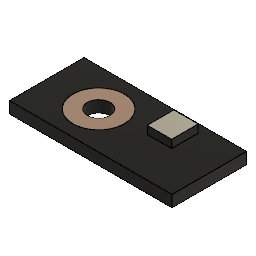
extruder_body_bltouch_190604 (Autodesk Fusion 360 archive; units mm, degrees)
design "filament_sensor"
Autodesk Fusion 360 part; units mm, degrees
sketch "Sketch1" plane through (0, 0, 0) normal (0, 0, 1) x (1, 0, 0)
  line L0 (0, 0) -> (22.2, 0)
  line L1 (22.2, 0) -> (22.2, 10.2)
  line L2 (22.2, 10.2) -> (0, 10.2)
  line L3 (0, 10.2) -> (0, 0)
  circle A0 centre (7.1, 5.1) radius 1.55
  line L4 (13.45, 9) -> (16.75, 9)
  line L5 (16.75, 9) -> (16.75, 5.4)
  line L6 (16.75, 5.4) -> (13.45, 5.4)
  line L7 (13.45, 5.4) -> (13.45, 9)
  circle A1 centre (7.1, 5.1) radius 3.5
  line L8 (15.1, 9) -> (15.1, 5.4) construction
  line L9 (11.15, 9.8) -> (13.25, 9.8)
  line L10 (13.25, 9.8) -> (13.25, 5.6)
  line L11 (13.25, 5.6) -> (11.15, 5.6)
  line L12 (11.15, 5.6) -> (11.15, 9.8)
  line L13 (12.2, 9.8) -> (12.2, 5.6) construction
  dimension "d1" = 22.2
  dimension "d2" = 10.2
  dimension "d3" = 3.1
  dimension "d4" = 7
  dimension "d5" = 8
  dimension "d6" = 3.3
  dimension "d7" = 3.6
  dimension "d8" = 5.1
  dimension "d9" = 7.1
  dimension "d10" = 1.2
  dimension "d11" = 0.4
  dimension "d12" = 2.1
  dimension "d13" = 4.2
  dimension "d14" = 5.1
  measures "d2" distance of L0.start
  measures "d3" diameter of A0
  measures "d4" diameter of A1
  measures "d6" distance of L5 L7
  measures "d8" distance of L2
  measures "d9" distance of L3
  measures "d10" distance of L2 L4
  measures "d11" distance of L2 L9
  measures "d12" distance of L10 L12
  measures "d14" distance of L13
extrude "Extrude1" add sketch "Sketch1" against normal blind 1.6 contours L0 L1 L2 L3 | L4 L5 L6 L7 | A1 | L9 L10 L11 L12
extrude "Extrude2" add sketch "Sketch1" along normal blind 0.01 contours A1
extrude "Extrude3" add sketch "Sketch1" along normal blind 1.1 contours L4 L5 L6 L7

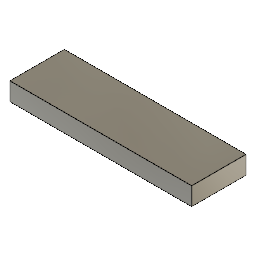
design "magnet_20x6x2"
Autodesk Fusion 360 part; units mm, degrees
sketch "Sketch1" plane through (0, 0, 0) normal (0, 0, 1) x (1, 0, 0)
  line L0 (0, 0) -> (20, 0)
  line L1 (20, 0) -> (20, 6)
  line L2 (20, 6) -> (0, 6)
  line L3 (0, 6) -> (0, 0)
  dimension "d1" = 6
  dimension "d2" = 20
  measures "d1" distance of L0.start
  measures "d2" distance of L0.start
extrude "Extrude1" add sketch "Sketch1" along normal blind 2

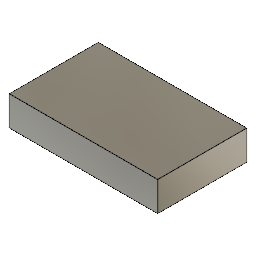
design "magnet_10x6x2"
Autodesk Fusion 360 part; units mm, degrees
sketch "Sketch1" plane through (0, 0, 0) normal (0, 0, 1) x (1, 0, 0)
  line L0 (0, 0) -> (10, 0)
  line L1 (10, 0) -> (10, 6)
  line L2 (10, 6) -> (0, 6)
  line L3 (0, 6) -> (0, 0)
  dimension "d1" = 10
  dimension "d2" = 6
  measures "d1" distance of L0.start
  measures "d2" distance of L0.start
extrude "Extrude1" add sketch "Sketch1" along normal blind 2

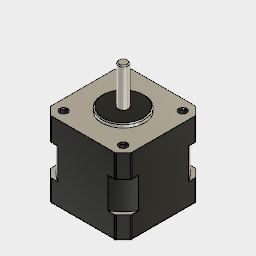
design "nema17_xye_ldo"
Autodesk Fusion 360 part; units mm, degrees
sketch "base" plane through (0, 0, 0) normal (0, 0, 1) x (1, 0, 0)
  line L0 (-21, -21) -> (21, -21)
  line L1 (21, -21) -> (21, 21)
  line L2 (21, 21) -> (-21, 21)
  line L3 (-21, 21) -> (-21, -21)
  line L4 (-21, -21) -> (21, 21) construction
  line L5 (21, -21) -> (-21, 21) construction
  circle A0 centre (0, 0) radius 11
  circle A1 centre (0, 0) radius 2.5
  circle A2 centre (-15.5, 15.5) radius 1.5
  circle A3 centre (15.5, 15.5) radius 1.5
  line L6 (-15.5, 15.5) -> (15.5, 15.5) construction
  circle A4 centre (15.5, -15.5) radius 1.5
  circle A5 centre (-15.5, -15.5) radius 1.5
  line L7 (-1.5, 2) -> (1.5, 2)
  dimension "d1" = 42
  dimension "d2" = 42
  dimension "d5" = 22
  dimension "d9" = 5
  dimension "d14" = 31
  dimension "d15" = 3
  dimension "d16" = 3
  dimension "d46" = 4.5
  measures "d1" distance of L0.end L1.end
  measures "d2" distance of L1.end L2.end
  measures "d5" diameter of A0
  measures "d9" diameter of A1
  measures "d14" distance of A2.centre A3.centre
  measures "d15" diameter of A2
  measures "d16" diameter of A3
extrude "Extrude1" add sketch "base" along normal blind 40 contours L0 L1 L2 L3 | A0 | A1 L7 | A1 L7 | A2 | A3 | A4 | A5 makes body 1
extrude "Extrude2" add sketch "base" along normal blind 2 from surface at 40 contours A0 | A1 L7 | A1 L7 bodies 1
extrude "Extrude3" add sketch "base" along normal blind 20 from surface at 42 contours A1 L7 picked at (0.6865, -0.2754) bodies 1
extrude "Extrude11" add sketch "base" along normal blind 1 from surface at 42 contours A1 L7 picked at (-0.3999, 2.0645) bodies 1
chamfer "Chamfer1" distance 4.2 angle 45 4 edges at (21, -21, 20) (21, 21, 20) (-21, 21, 20) (-21, -21, 20) on bodies 1
extrude "Extrude4" cut sketch "base" against normal blind 4.5 from surface at 40 contours A2 | A3 | A4 | A5 bodies 1
chamfer "Chamfer3" distance 0.5 angle 45 1 edges at (0, -2.5, 62) on bodies 1
chamfer "Chamfer4" distance 0.5 angle 45 1 edges at (-10.2556, -3.9778, 42) on bodies 1
sketch "core_shape" plane through (0, 0, 0) normal (0, 0, -1) x (1, 0, 0)
  line L0 (-16.8, 21) -> (-21, 16.8)
  line L1 (-21, 16.8) -> (-21, -16.8)
  line L2 (-21, -16.8) -> (-16.8, -21)
  line L3 (-16.8, -21) -> (16.8, -21)
  line L4 (16.8, -21) -> (21, -16.8)
  line L5 (21, -16.8) -> (21, 16.8)
  line L6 (21, 16.8) -> (16.8, 21)
  line L7 (16.8, 21) -> (-16.8, 21)
  circle A0 centre (0, 0) radius 24.7286
  line L8 (16.8, 21) -> (21, 16.8)
  arc A1 (1.5, -2) -> (-1.5, -2) centre (0, 0) ccw
  dimension "d31" = 2
  measures "d31" distance of A0 L8
extrude "Extrude6" cut sketch "core_shape" against normal up to surface (16 mm away) from surface at -12 contours L0 L1 L7 A0 | L5 L6 L7 A0 L8 | L1 L2 L3 A0 | L3 L4 L5 A0 bodies 1
sketch "back" plane through (0, 0, 0) normal (0, 0, -1) x (1, 0, 0)
  line L0 (-16.8, 21) -> (-21, 16.8)
  line L1 (-21, 16.8) -> (-21, -16.8)
  line L2 (-21, -16.8) -> (-16.8, -21)
  line L3 (-16.8, -21) -> (16.8, -21)
  line L4 (16.8, -21) -> (21, -16.8)
  line L5 (21, -16.8) -> (21, 16.8)
  line L6 (21, 16.8) -> (16.8, 21)
  line L7 (16.8, 21) -> (-16.8, 21)
  circle A0 centre (0, 0) radius 10.5
  circle A1 centre (0, 0) radius 3.479
  circle A2 centre (-15.5, 15.5) radius 1.5
  circle A3 centre (15.5, 15.5) radius 1.5
  circle A4 centre (-15.5, -15.5) radius 1.5
  circle A5 centre (15.5, -15.5) radius 1.5
  circle A6 centre (-15.5, 15.5) radius 3
  circle A7 centre (-15.5, -15.5) radius 3
  circle A8 centre (15.5, -15.5) radius 3
  circle A9 centre (15.5, 15.5) radius 3
  circle A10 centre (-15.5, 15.5) radius 2.6
  circle A11 centre (15.5, 15.5) radius 2.6
  circle A12 centre (-15.5, -15.5) radius 2.6
  circle A13 centre (15.5, -15.5) radius 2.6
  dimension "d50" = 6.958
  dimension "d58" = 6
  dimension "d59" = 6
  dimension "d60" = 6
  dimension "d61" = 6
  dimension "d62" = 5.2
  dimension "d63" = 5.2
  dimension "d64" = 5.2
  dimension "d65" = 5.2
  measures "d50" diameter of A1
  measures "d58" diameter of A6
  measures "d59" diameter of A7
  measures "d60" diameter of A8
  measures "d61" diameter of A9
  measures "d62" diameter of A10
  measures "d63" diameter of A11
  measures "d64" diameter of A12
  measures "d65" diameter of A13
extrude "Extrude8" cut sketch "back" against normal blind 2 contours A1 bodies 1
fillet "Fillet3" radius 0.2 1 edges at (-3.2436, -1.2581, 0) on bodies 1
extrude "Extrude10" cut sketch "back" against normal blind 4 contours A6 bodies 1
fillet "Fillet4" radius 1 1 edges at (-17.9241, -14.5598, 0) on bodies 1
pattern_circular "C-Pattern1" count 4 over 360 about axis through (0, 0, 1.75) along (0, 0, 1) of "Extrude10", "Fillet4"
sketch "cables" plane through (0, 21, 0) normal (0, 1, 0) x (-1, 0, 0)
  line L0 (-16.8, 0) -> (16.8, 0)
  circle A0 centre (0.75, 1.35) radius 0.75
  circle A1 centre (-0.75, 1.35) radius 0.75
  line L1 (-0.75, 1.35) -> (0.75, 1.35) construction
  line L2 (0.75, 1.35) -> (0.75, 0) construction
  line L3 (-0.75, 1.35) -> (-0.75, 2.85) construction
  line L4 (-0.75, 2.85) -> (0.75, 2.85) construction
  line L5 (0.75, 2.85) -> (0.75, 1.35) construction
  circle A2 centre (-0.75, 2.85) radius 0.75
  circle A3 centre (0.75, 2.85) radius 0.75
  line L6 (-3.5, 0) -> (3.5, 0)
  line L7 (3.5, 0) -> (3.5, 4)
  line L8 (3.5, 4) -> (-3.5, 4)
  line L9 (-3.5, 4) -> (-3.5, 0)
  line L10 (16.8, 0) -> (-16.8, 0)
  line L11 (-3.5, 0.3) -> (3.5, 0.3)
  dimension "d23" = 1.5
  dimension "d25" = 1.35
  dimension "d27" = 0.75
  dimension "d30" = 1.5
  dimension "d38" = 7
  dimension "d39" = 3.5
  dimension "d40" = 4
  dimension "d45" = 0.3
  measures "d23" diameter of A1
  measures "d25" distance of A0.centre L2.end
  measures "d27" distance of origin L2.end
  measures "d30" distance of A1.centre L2.end
  measures "d38" distance of L6.start L6.end
  measures "d39" distance of origin L6.end
  measures "d40" distance of L6.start L8.end
  measures "d45" distance of L6.end L11.end
extrude "Extrude5" add sketch "cables" along normal blind 5 separate body contours A0 | A1 | A3 | A2 makes body 2
extrude "Extrude7" add sketch "cables" along normal blind 0.3 and the other way blind 1.3 contours L7 L8 L9 L11 | A0 A1 A2 A3 | A3 | A2 bodies 1 2
fillet "Fillet1" radius 1 24 edges at (-21, 0, 0) (-18.9, -18.9, 0) (0, -21, 0) (-18.9, 18.9, 0) (0, 21, 0) (18.9, 18.9, 0) (21, 0, 0) (18.9, -18.9, 0) (-21, -16.8, 34) (-16.8, -21, 34) (-16.8, -21, 6) (-21, -16.8, 6) (-21, 16.8, 6) (-16.8, 21, 6) (-21, 16.8, 34) (-16.8, 21, 34) (16.8, 21, 34) (16.8, 21, 6) (21, 16.8, 34) (21, 16.8, 6) (21, -16.8, 6) (16.8, -21, 6) (16.8, -21, 34) (21, -16.8, 34) on bodies 1
chamfer "Chamfer2" distance 0.6 angle 45 4 edges at (14.1015, 16.0424, 40) (14.1015, -14.9576, 40) (-16.8985, -14.9576, 40) (-16.8985, 16.0424, 40) on bodies 1
equation "d26 = d23"
equation "d27 = d30 / 2"
equation "d30 = d23"
equation "d39 = d38 / 2"
equation "d59 = d58"
equation "d60 = d58"
equation "d61 = d58"
equation "d63 = d62"
equation "d64 = d62"
equation "d65 = d62"

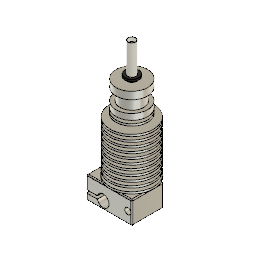
design "e3d_v6"
Autodesk Fusion 360 part; units mm, degrees
sketch "sink" plane through (0, 0, 0) normal (0, 0, 1) x (1, 0, 0) in component "sink"
  circle A0 centre (0, 0) radius 11.15
  circle A1 centre (0, 0) radius 6.4
  circle A2 centre (0, 0) radius 11
  dimension "d1" = 22.3
  dimension "d4" = 12.8
  dimension "d7" = 22
  dimension "d131" = 0
  dimension "d132" = 0
  dimension "d133" = 0
  dimension "d134" = 0
  dimension "d180" = 0
  dimension "d181" = 0
  dimension "d182" = 0
  dimension "d183" = 0
  dimension "d192" = 0
  dimension "d193" = 0
  dimension "d194" = 0
  dimension "d195" = 0
  constraint coincident A0.centre A1.centre
  constraint concentric A0 A1
  constraint concentric A1 A2
  measures "d1" diameter of A0
  measures "d4" diameter of A1
  measures "d7" diameter of A2
extrude "Extrude1" add sketch "sink" along normal blind 1 contours A0 | A1 | A2 makes body 1 in component "sink"
extrude "Extrude2" add sketch "sink" along normal blind 30 draft -3.6 contours A1 bodies 1 in component "sink"
extrude "Extrude3" add sketch "sink" along normal blind 1 from surface at 2.5 contours A1 | A2 bodies 1 in component "sink"
pattern_linear "R-Pattern1" count 10 spacing 2.5 along (0, 0, 1) of "Extrude3" in component "sink"
sketch "groove" plane through (0, 0, 30) normal (0, 0, 1) x (-1, 0, 0) in component "sink"
  circle A0 centre (0, 0) radius 4.5126
  circle A1 centre (0, 0) radius 4.5126
  circle A2 centre (0, 0) radius 8
  circle A3 centre (0, 0) radius 6
  dimension "d15" = 16
  dimension "d16" = 12
  constraint concentric A1 A2
  constraint concentric A2 A3
  measures "d15" diameter of A2
  measures "d16" diameter of A3
extrude "Extrude4" add sketch "groove" along normal blind 1 from surface at -2.5 contours A0 A1 | A2 | A3 bodies 1 in component "sink"
extrude "Extrude5" add sketch "groove" along normal blind 3 contours A0 A1 | A2 | A3 bodies 1 in component "sink"
extrude "Extrude6" add sketch "groove" along normal blind 6 from surface at 3 contours A0 A1 | A3 bodies 1 in component "sink"
extrude "Extrude7" add sketch "groove" along normal blind 3.7 from surface at 9 contours A0 A1 | A2 | A3 bodies 1 in component "sink"
sketch "top" plane through (0, 0, 42.7) normal (0, 0, 1) x (-1, 0, 0) in component "sink"
  circle A0 centre (0, 0) radius 8
  circle A1 centre (0, 0) radius 8
  circle A2 centre (0, 0) radius 3.5
  circle A3 centre (0, 0) radius 2.1
  circle A4 centre (0, 0) radius 2.5
  circle A5 centre (0, 0) radius 4
  dimension "d28" = 7
  dimension "d29" = 4.2
  dimension "d124" = 5
  dimension "d147" = 8
  constraint concentric A1 A2
  constraint concentric A2 A3
  constraint concentric A3 A4
  constraint concentric A4 A5
  measures "d28" diameter of A2
  measures "d29" diameter of A3
  measures "d124" diameter of A4
  measures "d147" diameter of A5
extrude "Extrude2'" cut sketch "top" against normal up to surface (42.7 mm away) contours A3 bodies 1 in component "sink"
extrude "Extrude3'" cut sketch "top" against normal blind 6.5 contours A2 | A4 | A5 bodies 1 in component "sink"
extrude "Extrude4'" cut sketch "top" against normal blind 2 draft -55 from surface at -6.5 contours A2 | A3 | A4 | A5 bodies 1 in component "sink"
extrude "Extrude5'" add sketch "top" against normal blind 6 contours A2 | A5 bodies 1 in component "sink"
extrude "Extrude8" add sketch "top" along normal blind 2 and the other way blind 5.5 contours A2 | A4 bodies 1 in component "sink"
extrude "Extrude1'" cut sketch "top" along normal blind 1 contours A2 bodies 1 in component "sink"
sketch "bottom" plane through (0, 0, 0) normal (0, 0, -1) x (1, 0, 0) in component "sink"
  circle A0 centre (0, 0) radius 2.1
  circle A1 centre (0, 0) radius 11.15
  circle A2 centre (0, 0) radius 3
  circle A3 centre (0, 0) radius 3.5
  dimension "d158" = 6
  dimension "d228" = 7
  constraint coincident A0.centre A1.centre
  constraint concentric A2 A3
  measures "d158" diameter of A2
  measures "d228" diameter of A3
extrude "Extrude6'" cut sketch "bottom" against normal blind 15.1 contours A0 | A2 bodies 1 in component "sink"
extrude "Extrude7'" cut sketch "bottom" against normal blind 2 draft -55 from surface at -15.1 contours A0 | A2 bodies 1 in component "sink"
extrude "Extrude8'" cut sketch "bottom" against normal blind 10.5 contours A3 bodies 1 in component "sink"
thread "Thread1" "ISO Metric profile 7.0 M7x1 6H" major diameter 7.1472 minor diameter 6.0355 pitch 1 angle 60 resizes the face on face at (3.4956, 0.1745, 7) on bodies 1 in component "sink"
sketch "Sketch4" plane through (0, 0, 0) normal (0, 0, 1) x (1, 0, 0) in component "ptfe"
  circle A0 centre (0, 0) radius 2
  circle A1 centre (0, 0) radius 1
  dimension "d168" = 4
  dimension "d169" = 2
  dimension "d176" = 0
  dimension "d177" = 0
  dimension "d178" = 0
  dimension "d179" = 0
  dimension "d188" = 0
  dimension "d189" = 0
  dimension "d190" = 0
  dimension "d191" = 0
  constraint coincident A0.centre A1.centre
  constraint concentric A0 A1
  measures "d168" diameter of A0
  measures "d169" diameter of A1
extrude "Extrude10" add sketch "Sketch4" along normal blind 50 separate body makes body 2 in component "ptfe"
chamfer "Chamfer2" distance 0.8 angle 60 1 edges at (-0.9323, 0.3616, 50) measured on face at (1.6555, -0.149, 50) on bodies 2 in component "ptfe"
chamfer "Chamfer3" distance 0.9 angle 45 1 edges at (-1.8647, -0.7232, 0) measured on face at (1.9901, -0.1991, 16.6667) on bodies 2 in component "ptfe"
sketch "Sketch1" plane through (0, 0, 0) normal (0, 0, 1) x (1, 0, 0) in component "break"
  circle A0 centre (0, 0) radius 1.48
  circle A1 centre (0, 0) radius 3
  circle A2 centre (0, 0) radius 3.5
  circle A3 centre (0, 0) radius 2.05
  circle A4 centre (0, 0) radius 1
  dimension "d37" = 2.96
  dimension "d75" = 6
  dimension "d82" = 0
  dimension "d83" = 0
  dimension "d84" = 0
  dimension "d85" = 0
  dimension "d196" = 7
  dimension "d197" = 4.1
  dimension "d198" = 2
  dimension "d235" = 0
  dimension "d236" = 0
  dimension "d237" = 0
  dimension "d238" = 0
  dimension "d243" = 0
  dimension "d244" = 0
  dimension "d245" = 0
  dimension "d246" = 0
  constraint coincident A0.centre A1.centre
  constraint concentric A0 A1
  constraint concentric A1 A2
  constraint concentric A3 A4
  measures "d37" diameter of A0
  measures "d75" diameter of A1
  measures "d196" diameter of A2
  measures "d197" diameter of A3
  measures "d198" diameter of A4
extrude "Extrude1''" add sketch "Sketch1" along normal blind 15 separate body contours A0 | A1 | A2 | A3 | A4 makes body 3 in component "break"
extrude "Extrude3''" cut sketch "Sketch1" along normal blind 4.5 contours A2 bodies 3 in component "break"
extrude "Extrude4''" cut sketch "Sketch1" along normal blind 4.4 contours A0 | A3 | A4 bodies 3 in component "break"
extrude "Extrude5''" cut sketch "Sketch1" along normal blind 20 contours A4 bodies 3 in component "break"
extrude "Extrude6''" add sketch "Sketch1" along normal blind 2.1 from surface at 15 contours A0 bodies 3 in component "break"
extrude "Extrude7''" add sketch "Sketch1" along normal blind 5 from surface at 17.1 contours A0 | A1 | A3 bodies 3 in component "break"
chamfer "Chamfer1" distance 0.5 angle 45 1 edges at (-0.9323, -0.3616, 4.4) measured on face at (1.6886, -0.1515, 4.4) on bodies 3 in component "break"
thread "Thread1'" "ISO Metric profile 7.0 M7x1 6g" major diameter 6.884 minor diameter 5.744 pitch 1 angle 60 resizes the face on face at (3.4826, -0.3485, 8) on bodies 3 in component "break"
thread "Thread2" "ISO Metric profile 6.0 M6x1 6g" major diameter 5.884 minor diameter 4.7435 pitch 1 angle 60 resizes the face on face at (2.9851, 0.2987, 20.4333) on bodies 3 in component "break"
chamfer "Chamfer2'" distance 0.5 angle 45 1 edges at (-2.7429, -1.0639, 22.1) on bodies 3 in component "break"
chamfer "Chamfer3'" distance 0.3 angle 45 1 edges at (-2.797, 1.0848, 0) on bodies 3 in component "break"
sketch "Sketch1 (2)" plane through (0, 0, 0) normal (0, 0, 1) x (1, 0, 0) in component "block"
  line L0 (0, 0) -> (23, 0)
  line L1 (23, 0) -> (23, 16)
  line L2 (23, 16) -> (0, 16)
  line L3 (0, 16) -> (0, 0)
  line L4 (0, 8) -> (23, 8) construction
  circle A0 centre (15, 8) radius 3
  circle A1 centre (2.5, 8) radius 1.5
  circle A2 centre (21, 8) radius 1.5
  dimension "d52" = 23
  dimension "d53" = 16
  dimension "d54" = 2
  dimension "d55" = 8
  dimension "d56" = 20.5
  dimension "d57" = 3
  dimension "d58" = 6
  dimension "d59" = 3
  dimension "d78" = 0
  dimension "d79" = 0
  dimension "d80" = 0
  dimension "d81" = 0
  dimension "d108" = 0
  dimension "d109" = 0
  dimension "d110" = 0
  dimension "d111" = 0
  dimension "d120" = 0
  dimension "d121" = 0
  dimension "d122" = 0
  dimension "d123" = 0
  dimension "d231" = 0
  dimension "d232" = 0
  dimension "d233" = 0
  dimension "d234" = 0
  dimension "d239" = 0
  dimension "d240" = 0
  dimension "d241" = 0
  dimension "d242" = 0
  dimension "d259" = 0
  dimension "d260" = 0
  dimension "d261" = 0
  dimension "d262" = 0
  constraint horizontal L0
  constraint vertical L1
  constraint horizontal L2
  constraint vertical L3
  constraint coincident L0.start L3.end
  constraint midpoint L3 L4.start
  constraint midpoint L1 L4.end
  constraint coincident L4 A0.centre
  constraint coincident L4 A1.centre
  constraint coincident L4 A2.centre
  measures "d52" horizontal distance of L1.end L2.end
  measures "d53" vertical distance of L0.start L2.end
  measures "d54" horizontal distance of L0.end A2.centre
  measures "d55" horizontal distance of L0.end A0.centre
  measures "d56" horizontal distance of L0.end A1.centre
  measures "d57" diameter of A1
  measures "d58" diameter of A0
  measures "d59" diameter of A2
extrude "Extrude1'''" add sketch "Sketch1 (2)" along normal blind 11.5 separate body contours L0 L1 L2 L3 | A2 makes body 4 in component "block"
sketch "Sketch2" plane through (0, 0, 0) normal (0, -1, 0) x (1, 0, 0) in component "block"
  line L0 (0, 0) -> (23, 0)
  line L1 (23, 0) -> (23, 11.5)
  line L2 (23, 11.5) -> (0, 11.5)
  line L3 (0, 11.5) -> (0, 0)
  circle A0 centre (21, 5.75) radius 1.55
  circle A1 centre (8.5, 4) radius 3
  line L4 (23, 0) -> (23, 11.5)
  line L5 (0, 0) -> (0, 11.5)
  line L6 (5.5953, 3.25) -> (0, 3.25)
  line L7 (5.5953, 4.75) -> (0, 4.75)
  line L8 (8.5, 4) -> (0, 4) construction
  dimension "d62" = 5.75
  dimension "d64" = 14.5
  dimension "d65" = 2
  dimension "d66" = 6
  dimension "d67" = 3.1
  dimension "d68" = 1.5
  dimension "d69" = 4
  constraint coincident A1 L6.start
  constraint coincident L5 L6.end
  constraint coincident A1 L7.start
  constraint coincident L5 L7.end
  constraint perpendicular L3 L6
  constraint perpendicular L3 L7
  constraint coincident A1.centre L8.start
  constraint coincident L5 L8.end
  constraint perpendicular L3 L8
  constraint symmetric L6 L7 L8
  measures "d62" vertical distance of L0.end A0.centre
  measures "d64" horizontal distance of L0.end A1.centre
  measures "d65" horizontal distance of L0.end A0.centre
  measures "d66" diameter of A1
  measures "d67" diameter of A0
  measures "d68" vertical distance of L6.end L7.end
  measures "d69" distance of L0.start L8
extrude "Extrude2''" cut sketch "Sketch2" against normal blind 29 contours L3 A1 L5 L6 L7 | A1 | A0 bodies 4 in component "block"
extrude "Extrude3'''" cut sketch "Sketch1 (2)" along normal blind 5.6 contours A2 bodies 4 in component "block"
fillet "Fillet1" radius 0.5 14 edges at (23, 0, 5.75) (23, 8, 11.5) (11.5, 0, 11.5) (11.5, 0, 0) (23, 8, 0) (11.5, 16, 0) (0, 8, 0) (0, 0, 1.625) (0, 0, 8.125) (0, 8, 11.5) (11.5, 16, 11.5) (23, 16, 5.75) (0, 16, 8.125) (0, 16, 1.625) on bodies 4 in component "block"
thread "Thread1''" "ISO Metric profile 6.0 M6x1 6H" major diameter 6.147 minor diameter 5.035 pitch 1 angle 60 resizes the face on face at (17.9963, 7.8505, 7.6667) on bodies 4 in component "block"
sketch "Sketch1 (3)" plane through (0, 0, 0) normal (0, 0, 1) x (1, 0, 0) in component "nozzle"
  circle A0 centre (0, 0) radius 3
  circle A1 centre (0, 0) radius 2.5
  circle A2 centre (0, 0) radius 3.5 construction
  line L0 (-3.5, -2.0207) -> (0, -4.0415)
  line L1 (0, -4.0415) -> (3.5, -2.0207)
  line L2 (3.5, -2.0207) -> (3.5, 2.0207)
  line L3 (3.5, 2.0207) -> (0, 4.0415)
  line L4 (0, 4.0415) -> (-3.5, 2.0207)
  line L5 (-3.5, 2.0207) -> (-3.5, -2.0207)
  circle A3 centre (0, 0) radius 1
  circle A4 centre (0, 0) radius 0.2
  dimension "d90" = 6
  dimension "d91" = 5
  dimension "d92" = 7
  dimension "d104" = 0
  dimension "d105" = 0
  dimension "d106" = 0
  dimension "d107" = 0
  dimension "d116" = 0
  dimension "d117" = 0
  dimension "d118" = 0
  dimension "d119" = 0
  dimension "d255" = 0
  dimension "d256" = 0
  dimension "d257" = 0
  dimension "d258" = 0
  dimension "d271" = 2
  dimension "d272" = 0.4
  constraint coincident A0.centre A1.centre
  constraint concentric A0 A1
  constraint concentric A1 A2
  constraint tangent A2 L5
  constraint vertical L5
  constraint concentric A3 A4
  measures "d90" diameter of A0
  measures "d91" diameter of A1
  measures "d92" diameter of A2
  measures "d271" diameter of A3
  measures "d272" diameter of A4
extrude "Extrude1''''" add sketch "Sketch1 (3)" along normal blind 6 separate body contours A0 | A1 | A3 makes body 5 in component "nozzle"
extrude "Extrude2'''" add sketch "Sketch1 (3)" along normal blind 7.5 contours A1 | A3 bodies 5 in component "nozzle"
extrude "Extrude3''''" add sketch "Sketch1 (3)" along normal blind 3 from surface at 7.5 contours A0 | A1 | L0 L1 L2 L3 L4 L5 | A3 bodies 5 in component "nozzle"
sketch "Sketch2 (2)" plane through (0, 0, 10.5) normal (0, 0, 1) x (-1, 0, 0) in component "nozzle"
  line L0 (0, -4.0415) -> (3.5, -2.0207)
  line L1 (3.5, -2.0207) -> (3.5, 2.0207)
  line L2 (3.5, 2.0207) -> (0, 4.0415)
  line L3 (0, 4.0415) -> (-3.5, 2.0207)
  line L4 (-3.5, 2.0207) -> (-3.5, -2.0207)
  line L5 (-3.5, -2.0207) -> (0, -4.0415)
  circle A0 centre (0, 0) radius 0.5
  circle A1 centre (0, 0) radius 0.2
  dimension "d100" = 1
  constraint coincident A0.centre A1.centre
  measures "d100" diameter of A0
extrude "Extrude4'''" add sketch "Sketch2 (2)" against normal blind 2 draft 30 from surface at 2 contours A0 | A1 bodies 5 in component "nozzle"
extrude "Extrude5'''" cut sketch "Sketch2 (2)" along normal up to surface (2 mm away) contours A1 bodies 5 in component "nozzle"
thread "Thread1'''" "ISO Metric profile 6.0 M6x1 6g" major diameter 5.884 minor diameter 4.7435 pitch 1 angle 60 resizes the face on face at (2.9963, -0.1495, 4) on bodies 5 in component "nozzle"
sketch "Sketch5" plane through (0, 0, 0) normal (1, 0, 0) x (0, 1, 0) in component "nozzle"
  line L0 (0.5, 12.5) -> (-0.5, 12.5)
  line L1 (1, 10.5144) -> (0.2, 11.9)
  line L2 (0.2, 11.9) -> (0, 11.9)
  line L3 (2.942, 0) -> (-2.942, 0)
  line L4 (1, 10.5144) -> (1, 0)
  line L5 (0, 12.5) -> (0, 0)
  point P0 (0, 12.5)
  dimension "d274" = 1
  dimension "d275" = 0.6
  dimension "d276" = 30
  dimension "d277" = 0.2
  constraint horizontal L2
  constraint coincident L3 L4.end
  constraint perpendicular L3 L4
  constraint coincident P0 L5.start
  constraint perpendicular L3 L5
  constraint coincident L2.end L5
  constraint coincident L5.end origin
  measures "d274" distance of L4 L5
  measures "d275" distance of L0 L2
  measures "d276" angle of L1 L5
  measures "d277" distance of L1.end L2.end
revolve "Revolve1" cut sketch "Sketch5" angle 360 about axis through (0, 0, 12.5) along (0, 0, -1) bodies 5 in component "nozzle"
chamfer "Chamfer2''" distance 0.3 angle 60 1 edges at (0.3616, -0.9323, 0) measured on face at (2.2828, 0.1711, 0) on bodies 5 in component "nozzle"
component "sink" placed x (1, 0, 0) y (0, 1, 0) z (0, 0, 1) at (0, 0, 0)
component "ptfe" placed x (1, 0, 0) y (0, 1, 0) z (0, 0, 1) at (0, 0, 9.6)
component "break" placed x (1, 0, 0) y (0, -1, 0) z (0, 0, -1) at (0, 0, 15)
component "block" placed x (1, 0, 0) y (0, 1, 0) z (0, 0, 1) at (-15, -8, -14.1)
component "nozzle" placed x (1, 0, 0) y (0, -1, 0) z (0, 0, -1) at (0, 0, -7)
equation "d37 = 2 mm + ( 0.48 * 2 ) * 1 mm"
equation "d187 = 50 mm - 32.1 mm - 1 mm"
equation "d274 = ( 2 / 2 ) * 1 mm"
equation "d276 = ( 60 / 2 ) * 1 deg"
equation "d277 = ( 0.4 / 2 ) * 1 mm"

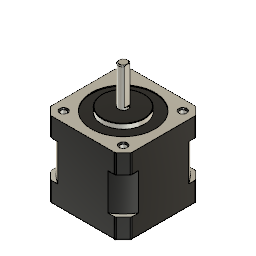
design "nema17_ldo_cool_power"
Autodesk Fusion 360 part; units mm, degrees
sketch "base" plane through (0, 0, 0) normal (0, 0, 1) x (1, 0, 0)
  line L0 (-21, -21) -> (21, -21)
  line L1 (21, -21) -> (21, 21)
  line L2 (21, 21) -> (-21, 21)
  line L3 (-21, 21) -> (-21, -21)
  line L4 (-21, -21) -> (21, 21) construction
  line L5 (21, -21) -> (-21, 21) construction
  circle A0 centre (0, 0) radius 11
  circle A1 centre (0, 0) radius 2.5
  circle A2 centre (-15.5, 15.5) radius 1.5
  circle A3 centre (15.5, 15.5) radius 1.5
  line L6 (-15.5, 15.5) -> (15.5, 15.5) construction
  circle A4 centre (15.5, -15.5) radius 1.5
  circle A5 centre (-15.5, -15.5) radius 1.5
  line L7 (2, 1.5) -> (2, -1.5)
  circle A6 centre (0, 0) radius 16.5
  dimension "d1" = 42
  dimension "d2" = 42
  dimension "d5" = 22
  dimension "d9" = 5
  dimension "d14" = 31
  dimension "d15" = 3
  dimension "d16" = 3
  dimension "d46" = 4.5
  dimension "d79" = 33
  constraint perpendicular L0 L1
  constraint parallel L0 L2
  constraint parallel L1 L3
  constraint horizontal L0
  constraint coincident L4 A0.centre
  constraint coincident L5 A0.centre
  constraint coincident A0.centre A1.centre
  constraint concentric A0 A1
  constraint coincident L5 A2.centre
  constraint coincident L4 A3.centre
  constraint coincident A2.centre L6.start
  constraint coincident A3.centre L6.end
  constraint parallel L2 L6
  constraint symmetric L4 A2 A4
  constraint symmetric L5 A3 A5
  constraint coincident A1 L7.start
  constraint coincident A1 L7.end
  constraint midpoint L4 A0.centre
  constraint vertical L7
  measures "d1" vertical distance of L0.end L1.end
  measures "d2" horizontal distance of L1.end L2.end
  measures "d5" diameter of A0
  measures "d9" diameter of A1
  measures "d14" horizontal distance of A2.centre A3.centre
  measures "d15" diameter of A2
  measures "d16" diameter of A3
  measures "d79" diameter of A6
extrude "Extrude1" add sketch "base" along normal blind 40 contours L0 L1 L2 L3 | A0 | A1 L7 | A1 L7 | A2 | A3 | A4 | A5 | A6
extrude "Extrude2" add sketch "base" along normal blind 2 from surface at 40 contours A0 | A1 L7 | A1 L7
extrude "Extrude3" add sketch "base" along normal blind 20 from surface at 42 contours A1 L7 picked at (-0.915, 0.4044)
extrude "Extrude11" add sketch "base" along normal blind 1 from surface at 42 contours A1 L7 picked at (2.1598, 0.107)
extrude "Extrude13" cut sketch "base" against normal blind 0.5 from surface at 40 contours A6
chamfer "Chamfer1" distance 4.2 angle 45 4 edges at (21, -21, 20) (21, 21, 20) (-21, 21, 20) (-21, -21, 20)
extrude "Extrude4" cut sketch "base" against normal blind 4.5 from surface at 40 contours A2 | A3 | A4 | A5
chamfer "Chamfer3" distance 0.5 angle 45 1 edges at (-2.5, 0, 62)
chamfer "Chamfer4" distance 0.2 angle 45 1 edges at (-10.2556, -3.9778, 42)
sketch "core_shape" plane through (0, 0, 0) normal (0, 0, -1) x (1, 0, 0)
  line L0 (-16.8, 21) -> (-21, 16.8)
  line L1 (-21, 16.8) -> (-21, -16.8)
  line L2 (-21, -16.8) -> (-16.8, -21)
  line L3 (-16.8, -21) -> (16.8, -21)
  line L4 (16.8, -21) -> (21, -16.8)
  line L5 (21, -16.8) -> (21, 16.8)
  line L6 (21, 16.8) -> (16.8, 21)
  line L7 (16.8, 21) -> (-16.8, 21)
  circle A0 centre (0, 0) radius 24.7286
  line L8 (16.8, 21) -> (21, 16.8)
  arc A1 (2, 1.5) -> (2, -1.5) centre (0, 0) ccw
  dimension "d31" = 2
  constraint coincident A0.centre A1.centre
  measures "d31" distance of A0 L8
extrude "Extrude6" cut sketch "core_shape" against normal up to surface (19 mm away) from surface at -11 contours L0 L1 L7 A0 | L5 L6 L7 A0 L8 | L1 L2 L3 A0 | L3 L4 L5 A0
sketch "back" plane through (0, 0, 0) normal (0, 0, -1) x (1, 0, 0)
  line L0 (-16.8, 21) -> (-21, 16.8)
  line L1 (-21, 16.8) -> (-21, -16.8)
  line L2 (-21, -16.8) -> (-16.8, -21)
  line L3 (-16.8, -21) -> (16.8, -21)
  line L4 (16.8, -21) -> (21, -16.8)
  line L5 (21, -16.8) -> (21, 16.8)
  line L6 (21, 16.8) -> (16.8, 21)
  line L7 (16.8, 21) -> (-16.8, 21)
  circle A0 centre (0, 0) radius 10.8
  circle A1 centre (0, 0) radius 4
  circle A2 centre (-15.5, 15.5) radius 1.5
  circle A3 centre (15.5, 15.5) radius 1.5
  circle A4 centre (-15.5, -15.5) radius 1.5
  circle A5 centre (15.5, -15.5) radius 1.5
  circle A6 centre (-15.5, 15.5) radius 3
  circle A7 centre (-15.5, -15.5) radius 3
  circle A8 centre (15.5, -15.5) radius 3
  circle A9 centre (15.5, 15.5) radius 3
  circle A10 centre (-15.5, 15.5) radius 2.6
  circle A11 centre (15.5, 15.5) radius 2.6
  circle A12 centre (-15.5, -15.5) radius 2.6
  circle A13 centre (15.5, -15.5) radius 2.6
  dimension "d50" = 8
  dimension "d58" = 6
  dimension "d59" = 6
  dimension "d60" = 6
  dimension "d61" = 6
  dimension "d62" = 5.2
  dimension "d63" = 5.2
  dimension "d64" = 5.2
  dimension "d65" = 5.2
  constraint concentric A0 A1
  constraint concentric A2 A6
  constraint concentric A4 A7
  constraint concentric A5 A8
  constraint concentric A3 A9
  constraint concentric A6 A10
  constraint concentric A9 A11
  constraint concentric A7 A12
  constraint concentric A5 A13
  measures "d50" diameter of A1
  measures "d58" diameter of A6
  measures "d59" diameter of A7
  measures "d60" diameter of A8
  measures "d61" diameter of A9
  measures "d62" diameter of A10
  measures "d63" diameter of A11
  measures "d64" diameter of A12
  measures "d65" diameter of A13
extrude "Extrude8" cut sketch "back" against normal blind 2 contours A1
extrude "Extrude12" cut sketch "back" against normal blind 0.5 draft -45 contours A2 | A3 | A4 | A5 | A6 | A7 | A8 | A9 | A10 | A11 | A12 | A13
sketch "cables" plane through (0, 21, 0) normal (0, 1, 0) x (-1, 0, 0)
  line L0 (-16.8, 0) -> (16.8, 0)
  circle A0 centre (1.25, 4) radius 0.75
  circle A1 centre (-1.25, 4) radius 0.75
  line L1 (-1.25, 4) -> (1.25, 4) construction
  line L2 (-1.25, 4) -> (-1.25, 6.5) construction
  line L3 (-1.25, 6.5) -> (1.25, 6.5) construction
  line L4 (1.25, 6.5) -> (1.25, 4) construction
  circle A2 centre (-1.25, 6.5) radius 0.75
  circle A3 centre (1.25, 6.5) radius 0.75
  line L5 (-4, 0) -> (4, 0)
  line L6 (4, 0) -> (4, 9)
  line L7 (4, 9) -> (-4, 9)
  line L8 (-4, 9) -> (-4, 0)
  line L9 (16.8, 0) -> (-16.8, 0)
  line L10 (-4, 2) -> (4, 2)
  line L11 (0, 4) -> (0, 0) construction
  dimension "d23" = 1.5
  dimension "d38" = 8
  dimension "d39" = 4
  dimension "d40" = 9
  dimension "d45" = 2
  dimension "d76" = 2
  dimension "d77" = 2.5
  dimension "d78" = 2.5
  constraint coincident A0.centre L1.end
  constraint coincident A1.centre L1.start
  constraint perpendicular L1 L2
  constraint perpendicular L3 L4
  constraint perpendicular L2 L3
  constraint coincident L2.end L3.start
  constraint coincident L3.end L4.start
  constraint horizontal L5
  constraint vertical L6
  constraint horizontal L7
  constraint vertical L8
  constraint coincident L0 L5.start
  constraint coincident L8 L10.start
  constraint coincident L6 L10.end
  constraint perpendicular L6 L10
  constraint midpoint L1 L11.start
  constraint coincident L11.end origin
  constraint perpendicular L5 L11
  constraint perpendicular L1 L11
  constraint equal A0 A1
  constraint equal A1 A3
  constraint equal A1 A2
  measures "d23" diameter of A1
  measures "d38" horizontal distance of L5.start L5.end
  measures "d39" horizontal distance of L11.end L5.end
  measures "d40" vertical distance of L5.start L7.end
  measures "d45" distance of L5.end L10.end
  measures "d76" vertical distance of A0.centre L10.end
  measures "d77" distance of A1.centre A0.centre
  measures "d78" distance of L3.end A0.centre
extrude "Extrude5" add sketch "cables" along normal blind 5 contours A0 | A1 | A2 | A3
extrude "Extrude7" add sketch "cables" along normal blind 0.3 and the other way blind 1.3 contours L6 L7 L8 L10 | A2 | A3
fillet "Fillet1" radius 1 24 edges at (-21, 0, 0) (-18.9, -18.9, 0) (0, -21, 0) (-18.9, 18.9, 0) (0, 21, 0) (18.9, 18.9, 0) (21, 0, 0) (18.9, -18.9, 0) (-21, -16.8, 35) (-16.8, -21, 35) (-16.8, -21, 5.5) (-21, -16.8, 5.5) (-21, 16.8, 5.5) (-16.8, 21, 5.5) (-21, 16.8, 35) (-16.8, 21, 35) (16.8, 21, 35) (16.8, 21, 5.5) (21, 16.8, 35) (21, 16.8, 5.5) (21, -16.8, 5.5) (16.8, -21, 5.5) (16.8, -21, 35) (21, -16.8, 35)
chamfer "Chamfer2" distance 0.6 angle 45 4 edges at (14.1015, 16.0424, 40) (14.1015, -14.9576, 40) (-16.8985, -14.9576, 40) (-16.8985, 16.0424, 40)
equation "d26 = d23"
equation "d30 = d23"
equation "d39 = d38 / 2"
equation "d59 = d58"
equation "d60 = d58"
equation "d61 = d58"
equation "d63 = d62"
equation "d64 = d62"
equation "d65 = d62"
equation "d77 = 1.5 mm + 1 mm"
equation "d78 = d77"

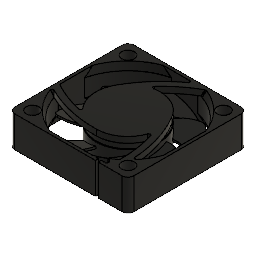
design "sunon_mf4010"
Autodesk Fusion 360 part; units mm, degrees
sketch "Sketch1" plane through (0, 0, 0) normal (0, 0, 1) x (1, 0, 0)
  line L0 (0, 0) -> (40, 0)
  line L1 (40, 0) -> (40, 40)
  line L2 (40, 40) -> (0, 40)
  line L3 (0, 40) -> (0, 0)
  line L4 (0, 20) -> (40, 20) construction
  circle A0 centre (20, 20) radius 19 construction
  circle A1 centre (4, 4) radius 2.1
  circle A2 centre (36, 4) radius 2.1
  line L5 (4, 4) -> (36, 4) construction
  circle A3 centre (4, 36) radius 2.1
  circle A4 centre (36, 36) radius 2.1
  circle A5 centre (20, 20) radius 10.75
  line L6 (29.1, 0) -> (29.1, 1)
  line L7 (29.1, 1) -> (27.4673, 1)
  line L8 (27.4673, 1) -> (31, 2.8)
  line L9 (31, 2.8) -> (31.8, 2)
  line L10 (31.8, 2) -> (31.8, 1)
  line L11 (31.8, 1) -> (30, 1)
  line L12 (30, 1) -> (30, 0)
  arc A6 (28.2838, 1.416) -> (28.3837, 1) centre (28.3837, 1.22) ccw
  arc A7 (31.2826, 2.5174) -> (30.644, 2.6186) centre (30.8937, 2.1285) ccw
  arc A8 (31.8, 1.7722) -> (31.6389, 2.1611) centre (31.25, 1.7722) ccw
  arc A9 (31.45, 1) -> (31.8, 1.35) centre (31.45, 1.35) ccw
  arc A10 (0, 2) -> (2, 0) centre (2, 2) ccw
  arc A11 (38, 0) -> (40, 2) centre (38, 2) ccw
  arc A12 (2, 40) -> (0, 38) centre (2, 38) ccw
  arc A13 (40, 38) -> (38, 40) centre (38, 38) ccw
  circle A14 centre (20, 20) radius 19.5
  line L13 (39, 24.3875) -> (39, 15.6125)
  line L14 (1, 24.3875) -> (1, 15.6125)
  line L15 (15.6125, 39) -> (24.3875, 39)
  line L16 (15.6125, 1) -> (24.3875, 1)
  circle A15 centre (4, 4) radius 2.85
  circle A16 centre (36, 4) radius 2.85
  circle A17 centre (36, 36) radius 2.85
  circle A18 centre (4, 36) radius 2.85
  arc A19 (-1.5, 15.2424) -> (20.1601, 9.2512) centre (19.5643, 49.2468) ccw
  arc A20 (-1.5, 17.6193) -> (13.0344, 11.812) centre (19.5643, 49.2468) ccw
  line L17 (-1.5, 15.2424) -> (-1.5, 17.6193)
  arc A21 (32.8117, 2.5708) -> (30.5738, 18.0616) centre (-5.1106, 4.9993) ccw
  line L18 (34.8702, 3.7592) -> (32.8117, 2.5708)
  arc A22 (34.8702, 3.7592) -> (29.2287, 25.5131) centre (-5.1106, 4.9993) ccw
  arc A23 (28.6883, 39.8099) -> (16.3918, 30.1264) centre (45.5463, 5.7539) ccw
  line L19 (26.6298, 40.9983) -> (28.6883, 39.8099)
  arc A24 (26.6298, 40.9983) -> (10.6112, 25.2357) centre (45.5463, 5.7539) ccw
  dimension "d1" = 40
  dimension "d2" = 40
  dimension "d3" = 1
  dimension "d4" = 32
  dimension "d5" = 4.2
  dimension "d6" = 4.2
  dimension "d8" = 4
  dimension "d9" = 4
  dimension "d10" = 21.5
  dimension "d19" = 0.9
  dimension "d20" = 10
  dimension "d21" = 1
  dimension "d22" = 27
  dimension "d23" = 1
  dimension "d24" = 135
  dimension "d25" = 1.8
  dimension "d26" = 1.8
  dimension "d27" = 0.22
  dimension "d28" = 0.55
  dimension "d29" = 0.35
  dimension "d30" = 0.55
  dimension "d32" = 2
  dimension "d33" = 2
  dimension "d34" = 2
  dimension "d35" = 2
  dimension "d43" = 39
  dimension "d45" = 5.7
  dimension "d46" = 5.7
  dimension "d47" = 5.7
  dimension "d48" = 5.7
  dimension "d91" = 40
  dimension "d92" = 2
  dimension "d99" = 360
  dimension "d101" = 9.5
  dimension "d102" = 1.5
  measures "d5" diameter of A1
  measures "d6" diameter of A2
  measures "d8" distance of L0.start
  measures "d9" distance of L0.start
  measures "d10" diameter of A5
  measures "d19" distance of L6 L12
  measures "d22" angle of L7 L8
  measures "d23" distance of L0.start
  measures "d24" angle of L9 L10
  measures "d26" distance of L10 L12
  measures "d27" radius of A6
  measures "d28" radius of A7
  measures "d29" radius of A9
  measures "d30" radius of A8
  measures "d32" radius of A10
  measures "d33" radius of A11
  measures "d34" radius of A12
  measures "d35" radius of A13
  measures "d43" diameter of A14
  measures "d45" diameter of A15
  measures "d46" diameter of A18
  measures "d47" diameter of A17
  measures "d48" diameter of A16
  measures "d91" radius of A19
  measures "d92" distance of A19 A20
  measures "d102" distance of L3 L17
extrude "Extrude1" add sketch "Sketch1" against normal blind 10.5 contours L0 L1 L2 L3 L6 L7 L8 L9 L10 L11 L12 A10 A11 A13 A14 A16 A19 A21 L18 A22 A23 L19 | L3 A14 A19 A20 | L2 L3 A12 A14 A20 A24 | L7 L8 A6 | A14 L14 A20 | A14 L14 A20 | A14 L16 | L10 L11 A9 | L8 L9 A7 | L2 A14 A23 L19 A24 | A14 L15 A24 | A14 A16 A21 L18 A22 | L9 L10 A8 | A14 L15 A24 | A14 L13 makes body 1
extrude "Extrude3" add sketch "Sketch1" against normal up to surface (10.5 mm away) contours A2 A16 L18 A22 | A2 A16 L18 A22 | A15 | A17 | A18 bodies 1
chamfer "Chamfer2" distance 0.8 distance2 2.3 4 edges at (6.2114, 6.2114, 0) (6.2114, 33.7886, 0) (33.7886, 33.7886, 0) (33.7886, 6.2114, 0) measured on face at (38.6989, 33.3592, 0) measured on face at (38.6989, 33.3592, 0) measured on face at (38.6989, 33.3592, 0) measured on face at (38.6989, 33.3592, 0) on bodies 1
chamfer "Chamfer3" distance 0.8 distance2 2.3 4 edges at (33.7886, 33.7886, -10.5) (6.2114, 33.7886, -10.5) (6.2114, 6.2114, -10.5) (33.7886, 6.2114, -10.5) measured on face at (38.6989, 33.3592, -10.5) measured on face at (38.6989, 33.3592, -10.5) measured on face at (38.6989, 33.3592, -10.5) measured on face at (38.6989, 33.3592, -10.5) on bodies 1
extrude "Extrude2" add sketch "Sketch1" against normal blind 2 contours L3 A14 A19 A20 | A5 A14 L14 A19 A20 | A14 L14 A20 | A5 | A5 A14 A21 A22 | L2 A14 A23 L19 A24 | A14 A16 A21 L18 A22 | A5 A14 L15 A23 A24 | A14 L15 A24 | A2 A16 L18 A22 picked at (0.9597, 15.9526) picked at (23.7523, 39.0599) picked at (34.5666, 5.9508) bodies 1
fillet "Fillet2" radius 0.5 9 edges at (13.0344, 11.812, -1) (30.5738, 18.0616, -1) (16.3918, 30.1264, -1) (34.8542, 6.6779, -0.9975) (1, 13.8156, -0.4583) (23.3044, 39, -1) (1, 16.0901, -1) (32.8887, 4.7695, -1.0002) (26.7446, 38.7766, -1.0029) on bodies 1
sketch "Sketch2" plane through (0, 0, -2) normal (0, 0, -1) x (1, 0, 0)
  arc A0 (17.9529, -30.5533) -> (29.2287, -25.5131) centre (20, -20) ccw
  line L0 (1, -15.1698) -> (1, -16.3845)
  line L1 (21.7147, -39) -> (24.8302, -39)
  circle A1 centre (20, -20) radius 10.45
  circle A2 centre (20, -20) radius 10.75
  arc A3 (24.8302, -39) -> (26.5926, -38.4626) centre (20, -20) ccw
  spline S0 degree 3 poles (26.1142, -38.4096) (26.1812, -38.4495) (26.2556, -38.4762) (26.3766, -38.4936) (26.4213, -38.4949) (26.5089, -38.4866) (26.5516, -38.4773) (26.5926, -38.4626) knots 0 0 0 0 0.023375 0.023375 0.036725 0.036725 0.049798 0.049798 0.049798 0.049798
  arc A4 (17.4886, -31.3813) -> (26.1142, -38.4096) centre (45.5463, -5.7539) ccw
  arc A5 (17.9529, -30.5533) -> (17.4886, -31.3813) centre (17.8577, -31.0441) ccw
  arc A6 (29.2287, -25.5131) -> (34.7377, -8.4794) centre (-5.1106, -4.9993) ccw
  spline S1 degree 3 poles (35.6194, -8.1525) (35.5794, -8.0997) (35.5299, -8.0548) (35.4202, -7.9911) (35.3626, -7.9712) (35.2449, -7.9561) (35.1867, -7.9602) (35.0717, -7.9906) (35.0166, -8.0177) (34.9126, -8.0944) (34.8662, -8.1454) (34.8038, -8.2443) (34.783, -8.2887) (34.752, -8.3816) (34.742, -8.4303) (34.7377, -8.4794) knots 0 0 0 0 0.019884 0.019884 0.038117 0.038117 0.055584 0.055584 0.073896 0.073896 0.094367 0.094367 0.108947 0.108947 0.123728 0.123728 0.123728 0.123728
  arc A7 (35.6194, -8.1525) -> (32.6928, -5.0594) centre (20, -20) ccw
  spline S2 degree 3 poles (32.8861, -5.5001) (32.8871, -5.4222) (32.873, -5.3444) (32.8276, -5.2309) (32.8064, -5.1916) (32.7554, -5.1199) (32.726, -5.0875) (32.6928, -5.0594) knots 0 0 0 0 0.023375 0.023375 0.036725 0.036725 0.049798 0.049798 0.049798 0.049798
  arc A8 (31.1123, -16.4843) -> (32.8861, -5.5001) centre (-5.1106, -4.9993) ccw
  arc A9 (30.163, -16.4962) -> (31.1123, -16.4843) centre (30.6356, -16.3332) ccw
  arc A10 (30.163, -16.4962) -> (20.1601, -9.2512) centre (20, -20) ccw
  arc A11 (20.1601, -9.2512) -> (1.723, -13.4461) centre (19.5643, -49.2468) ccw
  arc A12 (1.5051, -13.4985) -> (1.723, -13.4461) centre (1.5, -12.9986) ccw
  arc A13 (1.5051, -13.4985) -> (1, -15.1698) centre (20, -20) ccw
  arc A14 (1.2591, -15.9463) -> (1, -16.3845) centre (1.5, -16.3845) ccw
  arc A15 (11.3992, -12.1343) -> (1.2591, -15.9463) centre (19.5643, -49.2468) ccw
  arc A16 (11.8841, -12.9505) -> (11.3992, -12.1343) centre (11.5066, -12.6227) ccw
  arc A17 (11.8841, -12.9505) -> (10.6112, -25.2357) centre (20, -20) ccw
  arc A18 (10.6112, -25.2357) -> (22.0089, -38.0957) centre (45.5463, -5.7539) ccw
  arc A19 (21.7147, -39) -> (22.0089, -38.0957) centre (21.7147, -38.5) ccw
  arc A20 (17.9529, -30.5533) -> (29.2287, -25.5131) centre (20, -20) ccw
  dimension "d60" = 0.3
  measures "d60" distance of A1 A2
extrude "Extrude4" add sketch "Sketch2" along normal blind 1.8 separate body contours A1 makes body 2
extrude "Extrude5" add sketch "Sketch2" along normal up to surface (6.2 mm away) from surface at 1.8 contours A0 A2 A10 A17 A20 | A1 bodies 2
ref_plane "WorkPlane1" through (20, 20, -7.05) normal (0.781831, 0.62349, 0) x (0, 0, -1)
sketch "Sketch4" plane through (20, 20, -7.05) normal (0.781831, 0.62349, 0) x (0, 0, -1)
  line L0 (2.95, 10.75) -> (2.95, -10.75)
  line L1 (-3.25, 10.75) -> (-3.25, -10.75)
  line L2 (2.95, -10.75) -> (-3.9162, 10.5351)
  line L3 (-3.25, 10.75) -> (2.95, -8.4699)
  line L4 (2.95, -9.61) -> (-3.25, 9.61) construction
  line L5 (-0.15, 0) -> (2.95, 0) construction
  line L6 (-3.9162, 10.5351) -> (-3.25, 10.75)
  dimension "d67" = 0.7
  measures "d67" distance of L2 L3
extrude "Extrude6" add sketch "Sketch4" along normal blind 18.7 bodies 2
sketch "Sketch3" plane through (0, 0, -10) normal (0, 0, -1) x (1, 0, 0)
  line L0 (39.9011, -25.0372) -> (27.9177, -40.0639)
  circle A0 centre (20, -20) radius 10.75
  line L1 (39.9011, -25.0372) -> (41.3228, -23.2546)
  line L2 (41.3228, -23.2546) -> (26.7025, -11.5953)
  line L3 (13.2975, -28.4047) -> (27.9177, -40.0639)
  arc A1 (24.633, -29.7004) -> (31.6492, -34.3717) centre (34.3678, -22.6837) ccw
  arc A2 (31.6492, -34.3717) -> (38.1398, -23.6326) centre (20, -20) ccw
  arc A3 (28.9138, -26.0088) -> (38.1398, -23.6326) centre (31.3338, -16.3061) ccw
  line L4 (30.4566, -17.5054) -> (39.9011, -25.0372)
  line L5 (33.9094, -32.5506) -> (27.6465, -27.556) construction
  line L6 (24.1769, -29.9053) -> (31.4155, -35.6779)
  arc A4 (24.3875, -39) -> (39, -24.3875) centre (20, -20) ccw
  circle A5 centre (20, -20) radius 10.45
  dimension "d82" = 12
  dimension "d84" = 4
  dimension "d85" = 0.5
  dimension "d86" = 2
  dimension "d87" = 10
  dimension "d105" = 1
  dimension "d107" = 0.3
  measures "d82" radius of A1
  measures "d87" radius of A3
  measures "d105" distance of A2 A4
  measures "d107" distance of A0 A5
extrude "Extrude7" cut sketch "Sketch3" against normal blind 8.5 contours A0 L1 L2 L4 | L0 A1 A2 L4 L6 | A0 A3 L4 | L0 A0 L3 L6 A4 | L0 L3 A4 | A0 A1 L6 bodies 2
extrude "Extrude8" cut sketch "Sketch3" against normal up to surface (1.8 mm away) from surface at -6.2 contours A0 bodies 2
fillet "Fillet4" radius 2 1 edges at (31.6492, 34.3717, -5.6184) on bodies 2
fillet "Fillet5" radius 0.2 1 edges at (38.1398, 23.6326, -9.6322) on bodies 2
pattern_circular "C-Pattern1" count 7 over 360 about axis through (20, 20, -0.55) along (0, 0, -1) of 7 faces at (29.6538, 33.719, -5.2646) (31.9481, 33.9923, -5.8974) (30.2555, 31.108, -5.7934) (37.641, 25.5719, -8.9164) (31.2917, 30.4851, -6.8944) (31.0531, 26.3021, -7.6607) (37.9606, 24.0436, -9.5918) on bodies 2
fillet "Fillet3" radius 0.8 1 edges at (9.9775, 16.1126, -10) on bodies 2
combine "Combine1" operation add target body 2 tool bodies 1
equation "d6 = d5"
equation "d8 = ( d2 - d4 ) / 2"
equation "d9 = ( d2 - d4 ) / 2"
equation "d30 = d28"
equation "d32 = d34"
equation "d33 = d34"
equation "d46 = d45"
equation "d47 = d45"
equation "d48 = d45"
equation "d61 = ( 360 / 7 ) * 1 deg"

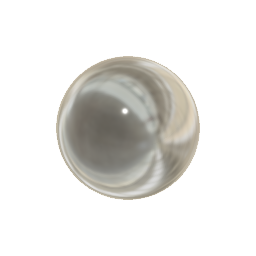
design "steel_ball"
Autodesk Fusion 360 part; units mm, degrees
sphere "SpherePrimitive1" add diameter 7 placed x (1, 0, 0) y (0, 1, 0) z (0, 0, 1) at (0, 0, 0)
